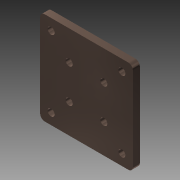
# Autodesk Inventor part: Topp
Saved by Autodesk Inventor 2015 (Build 190159000, 159)
## iProperties
Created: 2017-01-12
Part Number: Topp
Material: Generic
Document SubType Name: Modeling
Designer: Per
Density: 1 g/cm^3
Appearance: Gunmetal
Author: Per
Autodesk Inventor part; units mm, degrees
ref_plane "YZ Plane" through (0, 0, 0) normal (1, 0, 0) x (0, 1, 0)
ref_plane "XZ Plane" through (0, 0, 0) normal (0, 1, 0) x (-1, 0, 0)
ref_plane "XY Plane" through (0, 0, 0) normal (0, 0, 1) x (1, 0, 0)
sketch "Sketch1" plane through (0, 0, 0) normal (0, 1, 0) x (-1, 0, 0)
  line L0 (0, 0) -> (-36, 0)
  line L1 (-36, 0) -> (-36, -36)
  line L2 (-36, -36) -> (0, -36)
  line L3 (0, -36) -> (0, 0)
  circle A0 centre (-10.5282, -25.3471) radius 1.5
  circle A1 centre (-25.4718, -25.3471) radius 1.5
  circle A2 centre (-10.5282, -10.6529) radius 1.5
  circle A3 centre (-25.4718, -10.6529) radius 1.5
  line L4 (2, -38) -> (2, 2)
  line L5 (2, 2) -> (-38, 2)
  line L6 (-38, 2) -> (-38, -38)
  line L7 (-38, -38) -> (2, -38)
  circle A4 centre (-2.75, -2.75) radius 1.5
  circle A5 centre (-33.25, -2.75) radius 1.5
  circle A6 centre (-33.25, -33.25) radius 1.5
  circle A7 centre (-2.75, -33.25) radius 1.5
  dimension "d0" = 36
  dimension "d1" = 36
  dimension "d50" = 40
  dimension "d51" = 40
  dimension "d55" = 3
  dimension "d56" = 3
  dimension "d57" = 3
  dimension "d58" = 3
  constraints: 16 end point, 8 centre point, 5 parallel, 2 perpendicular, 1 horizontal
  measures "d0" distance of L2.end L1.end
  measures "d1" distance of L1.end L0.end
  measures "d50" distance of L4.start L4.end
  measures "d51" distance of L5.end L4.end
  measures "d55" diameter of A4
  measures "d56" diameter of A5
  measures "d57" diameter of A6
  measures "d58" diameter of A7
extrude "Extrusion3" add sketch "Sketch1" along normal blind 3 contours L3 L2 L1 L0 | L7 L6 L5 L4
fillet "Fillet2" radius 2 4 edges at (38, 1.5, 2) (-2, 1.5, 2) (-2, 1.5, -38) (38, 1.5, -38)
body "Solid3"
